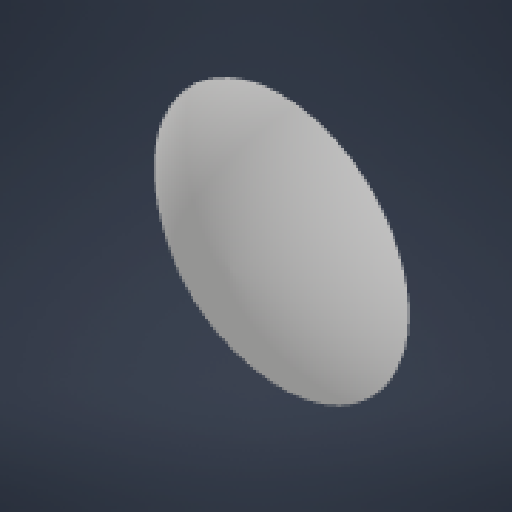
# Autodesk Inventor part: Central_spinner_cap
Saved by Autodesk Inventor 2026 (Build 300175050, 175E)
## iProperties
Created: 2026-05-09
Part Number: Central_spinner_cap
Material: Generic
Document SubType Name: Modeling
Designer: sniel
Density: 1 g/cm^3
Appearance: Default
Author: sniel
Autodesk Inventor part; units mm, degrees
ref_plane "YZ Plane" through (0, 0, 0) normal (1, 0, 0) x (0, 1, 0)
ref_plane "XZ Plane" through (0, 0, 0) normal (0, 1, 0) x (-1, 0, 0)
ref_plane "XY Plane" through (0, 0, 0) normal (0, 0, 1) x (1, 0, 0)
sketch "Sketch1" plane through (0, 0, 0) normal (1, 0, 0) x (0, 1, 0)
  line L0 (7.5, 0) -> (-7.5, 0)
  line L1 (7.5, -4) -> (7.5, 0)
  line L2 (17.5, -4) -> (-17.5, -4)
  line L3 (0, 0) -> (0, 3)
  arc A0 (17.5, -4) -> (0, 3) centre (-1.1618, -25.2794) ccw
  line L4 (0, -31.2352) -> (0, 10.4553) projected
  dimension "d0" = 3
  constraints: 8 end point, 2 point on circle, 1 centre point, 1 vertical
  measures "d0" distance of L3.start L3.end
revolve "Revolution1" add sketch "Sketch1" angle 360 about axis through (0, 0, -10) along (0, 0, 1) contours L0 L3 A0 L2 L1
body "Solid1"
